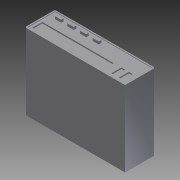
# Autodesk Inventor part: AbstractBox
Saved by Autodesk Inventor 2012 (Build 160160000, 160)
## iProperties
Created: 2013-07-09
Part Number: AbstractBox
Material: Default
Document SubType Name: Modeling
Designer: 1
Density: 1 g/cm^3
Author: 1
Autodesk Inventor part; units mm, degrees
ref_plane "YZ Plane" through (0, 0, 0) normal (1, 0, 0) x (0, 1, 0)
ref_plane "XZ Plane" through (0, 0, 0) normal (0, 1, 0) x (-1, 0, 0)
ref_plane "XY Plane" through (0, 0, 0) normal (0, 0, 1) x (1, 0, 0)
sketch "Sketch1" plane through (0, 0, 0) normal (0, 0, 1) x (1, 0, 0)
  line L0 (-50, -180) -> (-450, -180)
  line L1 (-450, -180) -> (-450, 120)
  line L2 (-450, 120) -> (-50, 120)
  line L3 (-50, 120) -> (-50, -180)
  point P0 (0, 0)
  dimension "d0" = 50
  dimension "d1" = 300
  dimension "d2" = 400
  dimension "d3" = 120
  constraints: 8 end point, 2 parallel, 1 horizontal, 1 perpendicular
  measures "d0" distance from line of L3 point (0, 0)
  measures "d1" distance between parallel lines of L0 L2
  measures "d2" distance of L1.end L2.end
  measures "d3" distance from line of point (0, 0) L2
extrude "Extrusion1" add sketch "Sketch1" along normal blind 120
sketch "Sketch2" plane through (-450, 120, 0) normal (0, 1, 0) x (1, 0, 0)
  line L0 (0, 0) -> (400, 0) projected
  line L1 (0, 0) -> (0, -120) projected
  line L2 (0, -120) -> (400, -120) projected
  line L3 (400, 0) -> (400, -120) projected
  line L4 (205, -30) -> (180, -30)
  line L5 (180, -30) -> (180, -20)
  line L6 (180, -20) -> (205, -20)
  line L7 (205, -20) -> (205, -30)
  dimension "d6" = 25
  dimension "d7" = 10
  dimension "d8" = 20
  dimension "d9" = 220
  constraints: 8 end point, 2 parallel, 1 horizontal, 1 perpendicular
  measures "d6" distance of L4.start L4.end
  measures "d7" distance of L4.end L5.end
  measures "d8" distance between parallel lines of L0 L6
  measures "d9" distance between parallel lines of L3 L5
extrude "Extrusion2" add sketch "Sketch2" along normal blind 10 contours L4 L5 L6 L7
pattern_linear "Rectangular Pattern1" count 4 spacing 50 along (-1, 0, 0) of "Extrusion2"
sketch "Sketch3" plane through (-450, 120, 0) normal (0, 1, 0) x (1, 0, 0)
  line L0 (0, -120) -> (400, -120) projected
  line L1 (400, 0) -> (400, -120) projected
  line L2 (0, 0) -> (400, 0) projected
  line L3 (0, 0) -> (0, -120) projected
  line L4 (15, -65) -> (300, -65)
  line L5 (300, -65) -> (300, -105)
  line L6 (300, -105) -> (15, -105)
  line L7 (15, -105) -> (15, -65)
  line L8 (330, -65) -> (345, -65)
  line L9 (345, -65) -> (345, -105)
  line L10 (345, -105) -> (330, -105)
  line L11 (330, -105) -> (330, -65)
  line L12 (360, -65) -> (375, -65)
  line L13 (375, -65) -> (375, -105)
  line L14 (375, -105) -> (360, -105)
  line L15 (360, -105) -> (360, -65)
  point P0 (450, 0)
  dimension "d15" = 65
  dimension "d16" = 15
  dimension "d17" = 15
  dimension "d18" = 100
  dimension "d21" = 30
  dimension "d22" = 15
  dimension "d23" = 15
  constraints: 24 end point, 6 parallel, 3 collinear, 3 horizontal, 3 perpendicular, 2 point on line
  measures "d15" distance between parallel lines of L2 L4
  measures "d16" distance between parallel lines of L0 L6
  measures "d17" distance between parallel lines of L3 L7
  measures "d18" distance between parallel lines of L1 L5
  measures "d21" distance between parallel lines of L5 L11
  measures "d22" distance between parallel lines of L15 L9
  measures "d23" distance of L8.start L8.end
extrude "Extrusion3" cut sketch "Sketch3" against normal blind 5 contours L4 L5 L6 L7 | L8 L9 L10 L11 | L12 L13 L14 L15
chamfer "Chamfer1" distance 4 angle 45 3 edges at (-450, -30, 120) (-450, -30, 0) (-50, -30, 0)
sketch "Sketch4" plane through (-446, 120, 0) normal (0, 1, 0) x (1, 0, 0)
  line L0 (392, 0) -> (396, -4) projected
  line L1 (0, 0) -> (392, 0) projected
  line L2 (-4, -4) -> (0, 0) projected
  line L3 (-4, -4) -> (-4, -116) projected
  line L4 (0, -120) -> (-4, -116) projected
  line L5 (0, -120) -> (396, -120) projected
  line L6 (396, -4) -> (396, -120) projected
  line L7 (389.8859, -5.1039) -> (390.8961, -6.1141)
  line L8 (390.8961, -6.1141) -> (390.8961, -114.8961)
  line L9 (390.8961, -114.8961) -> (2.1141, -114.8961)
  line L10 (2.1141, -114.8961) -> (1.1039, -113.8859)
  line L11 (1.1039, -113.8859) -> (1.1039, -6.1141)
  line L12 (1.1039, -6.1141) -> (2.1141, -5.1039)
  line L13 (2.1141, -5.1039) -> (389.8859, -5.1039)
  point P0 (446, 0)
  constraints: 14 end point, 6 other
extrude "Extrusion4" add sketch "Sketch4" along normal blind 2
body "Solid1"
